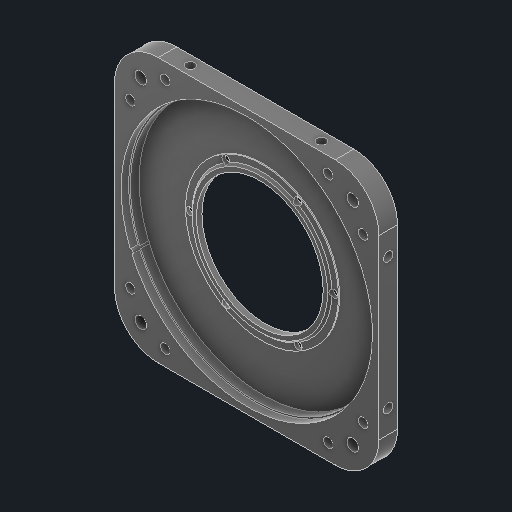
# Autodesk Inventor part: stator_center_01_back_p
Saved by Autodesk Inventor 2026.1 (Build 301233000, 233)
## iProperties
Created: 2026-04-12
Part Number: stator_center_01_back_p
Material: PC/ABS Plastic
Document SubType Name: Modeling
Designer: aaron
Density: 1.1 g/cm^3
Appearance: Smooth - White
Author: aaron
Autodesk Inventor part; units mm, degrees
ref_plane "YZ Plane" through (0, 0, 0) normal (1, 0, 0) x (0, 1, 0)
ref_plane "XZ Plane" through (0, 0, 0) normal (0, 1, 0) x (-1, 0, 0)
ref_plane "XY Plane" through (0, 0, 0) normal (0, 0, 1) x (1, 0, 0)
sketch "Sketch1" plane through (0, 0, 0) normal (0, 0, 1) x (1, 0, 0)
  circle A0 centre (0, 0) radius 57.5
  circle A1 centre (0, 0) radius 60.5
  line L0 (-40.5, 60.5) -> (40.5, 60.5)
  line L1 (60.5, 40.5) -> (60.5, -40.5)
  line L2 (40.5, -60.5) -> (-40.5, -60.5)
  line L3 (-60.5, -40.5) -> (-60.5, 40.5)
  arc A2 (-40.5, 60.5) -> (-60.5, 40.5) centre (-40.5, 40.5) ccw
  arc A3 (60.5, 40.5) -> (40.5, 60.5) centre (40.5, 40.5) ccw
  arc A4 (40.5, -60.5) -> (60.5, -40.5) centre (40.5, -40.5) ccw
  arc A5 (-60.5, -40.5) -> (-40.5, -60.5) centre (-40.5, -40.5) ccw
  dimension "d0" = 115
  dimension "d1" = 121
  dimension "d2" = 20
  constraints: 12 tangent, 8 end point, 8 point on circle, 6 centre point, 3 equal radius, 2 coincident, 2 parallel, 1 horizontal, 1 perpendicular
  measures "d0" diameter of A0
  measures "d1" diameter of A1
  measures "d2" radius of A2
extrude "Extrusion1" add sketch "Sketch1" along normal blind 7.5
sketch "Sketch3" plane through (0, 0, 7.5) normal (0, 0, 1) x (1, 0, 0)
  circle A0 centre (-48.4934, -48.5066) radius 2.65 projected
  circle A1 centre (-37.2752, -53.25) radius 2.15 projected
  circle A2 centre (-53.2398, -37.2897) radius 2.15 projected
  circle A3 centre (-53.25, 37.2752) radius 2.15 projected
  circle A4 centre (-48.5066, 48.4934) radius 2.65 projected
  circle A5 centre (-37.2897, 53.2398) radius 2.15 projected
  circle A6 centre (53.2398, 37.2897) radius 2.15 projected
  circle A7 centre (48.4934, 48.5066) radius 2.65 projected
  circle A8 centre (37.2752, 53.25) radius 2.15 projected
  circle A9 centre (53.25, -37.2752) radius 2.15 projected
  circle A10 centre (48.5066, -48.4934) radius 2.65 projected
  circle A11 centre (37.2897, -53.2398) radius 2.15 projected
  point P0 (0, 0)
extrude "Extrusion3" cut sketch "Sketch3" against normal through all
sketch "Sketch4" plane through (0, 0, 0) normal (0, 0, -1) x (-1, 0, 0)
  circle A0 centre (53.2398, -37.2897) radius 2.15 projected
  circle A1 centre (-53.2398, 37.2897) radius 2.15 projected
  circle A2 centre (-48.5066, -48.4934) radius 2.65 projected
  circle A3 centre (-37.2897, -53.2398) radius 2.15 projected
  circle A4 centre (37.2897, 53.2398) radius 2.15 projected
  circle A5 centre (48.4934, -48.5066) radius 2.65 projected
  circle A6 centre (53.25, 37.2752) radius 2.15 projected
  circle A7 centre (-48.4934, 48.5066) radius 2.65 projected
  circle A8 centre (-53.25, -37.2752) radius 2.15 projected
  circle A9 centre (-37.2752, 53.25) radius 2.15 projected
  circle A10 centre (48.5066, 48.4934) radius 2.65 projected
  circle A11 centre (37.2752, -53.25) radius 2.15 projected
  line L0 (60.5, 40.5) -> (60.5, -40.5) projected
  arc A12 (60.5, 40.5) -> (40.5, 60.5) centre (40.5, 40.5) ccw projected
  line L1 (-40.5, 60.5) -> (40.5, 60.5) projected
  arc A13 (-40.5, 60.5) -> (-60.5, 40.5) centre (-40.5, 40.5) ccw projected
  line L2 (-60.5, -40.5) -> (-60.5, 40.5) projected
  arc A14 (-60.5, -40.5) -> (-40.5, -60.5) centre (-40.5, -40.5) ccw projected
  line L3 (40.5, -60.5) -> (-40.5, -60.5) projected
  arc A15 (40.5, -60.5) -> (60.5, -40.5) centre (40.5, -40.5) ccw projected
  circle A16 centre (0, 0) radius 57.5 projected
  circle A17 centre (0, 0) radius 29
  dimension "d28" = 58
  constraints: 1 centre point, 1 coincident
  measures "d28" diameter of A17
extrude "Extrusion4" add sketch "Sketch4" along normal blind 1 contours L0 A15 L3 A14 L2 A13 L1 A12 | A16
sketch "Sketch5" plane through (0, 0, 0) normal (0, 0, 1) x (1, 0, 0)
  circle A0 centre (0, 0) radius 57.5 projected
  circle A1 centre (0, 0) radius 56.75
  dimension "d31" = 113.5
  constraints: 1 centre point, 1 coincident
  measures "d31" diameter of A1
extrude "Extrusion5" add sketch "Sketch5" along normal blind 4
sketch "Sketch6" plane through (0, 0, 0) normal (0, 0, 1) x (1, 0, 0)
  circle A0 centre (0, 0) radius 29 projected
  circle A1 centre (0, 0) radius 35
  dimension "d34" = 6
  constraints: 1 centre point
  measures "d34" radial gap between concentric circles of A0 A1
extrude "Extrusion6" add sketch "Sketch6" along normal blind 0.5
sketch "Sketch7" plane through (0, 0, 0.5) normal (0, 0, 1) x (1, 0, 0)
  circle A0 centre (0, 0) radius 29 projected
  circle A1 centre (0, 0) radius 31
  dimension "d37" = 2
  constraints: 1 centre point
  measures "d37" radial gap between concentric circles of A0 A1
extrude "Extrusion7" add sketch "Sketch7" along normal blind 1
chamfer "Chamfer1" distance 1 angle 45 1 edges at (-31, 0, 0.5)
sketch "Sketch8" plane through (0, 0, -1) normal (0, 0, -1) x (-1, 0, 0)
  circle A0 centre (32.9998, -0.1078) radius 1.65 projected
  circle A1 centre (0, 0) radius 29 projected
  circle A2 centre (32.9998, -0.1078) radius 1.75
  circle A3 centre (16.5932, 28.5248) radius 1.75
  circle A4 centre (-16.4066, 28.6326) radius 1.75
  circle A5 centre (-32.9998, 0.1078) radius 1.75
  circle A6 centre (-16.5932, -28.5248) radius 1.75
  circle A7 centre (16.4066, -28.6326) radius 1.75
  point P0 (0, 0)
  dimension "d43" = 3.5
  dimension "d46" = 360
  constraints: 6 centre point, 1 coincident, 13 other
  measures "d43" diameter of A2
extrude "Extrusion8" cut sketch "Sketch8" against normal through all contours A0 | A2 | A3 | A4 | A5 | A6 | A7
sketch "Sketch10" plane through (0, 0, 7.5) normal (0, 0, 1) x (1, 0, 0)
  arc A0 (-52.5046, -23.4417) -> (-51.9843, -22.1333) centre (-52.9044, -22.525) ccw projected
  arc A1 (-51.9843, -22.1333) -> (-53.2881, -21.6016) centre (-52.9044, -22.525) ccw projected
  circle A2 centre (-52.9044, -22.525) radius 0.9
  point P0 (0, 0)
  dimension "d50" = 1.8
  constraints: 1 centre point, 1 coincident
  measures "d50" diameter of A2
extrude "Extrusion9" add sketch "Sketch10" against normal up to surface (7.5 mm away)
sketch "Sketch11" plane through (-40.5, 60.5, 7.5) normal (0, 1, 0) x (1, 0, 0)
  line L0 (5.3603, 0) -> (5.3603, 8.5) projected
  line L1 (75.6252, 0) -> (75.6252, 8.5) projected
  circle A0 centre (40.5, 4.25) radius 2.15
  line L2 (101, 8.5) -> (101, 0) projected
  line L3 (-20, 0) -> (-20, 8.5) projected
  line L4 (-20, 0) -> (0, 0) projected
  line L5 (0, 8.5) -> (-20, 8.5) projected
  circle A1 centre (10.5, 4.25) radius 2.15
  circle A2 centre (70.5, 4.25) radius 2.15
  point P0 (40.5, 7.5)
  dimension "d53" = 4.3
  dimension "d54" = 121
  dimension "d55" = 8.5
  dimension "d56" = 60.5
  dimension "d57" = 4.25
  dimension "d60" = 30
  dimension "d67" = 30
  constraints: 3 centre point, 2 horizontal, 4 other
  measures "d53" diameter of A0
  measures "d54" distance between parallel lines of L2 L3
  measures "d55" distance between parallel lines of L4 L5
  measures "d56" distance from line of L3 A0.centre
  measures "d57" distance from line of L5 A0.centre
  measures "d60" distance of A0.centre A1.centre
  measures "d67" distance of A0.centre A2.centre
extrude "Extrusion10" cut sketch "Sketch11" against normal blind 10 contours A1 | A2
sketch "Sketch12" plane through (-40.5, -60.5, 7.5) normal (0, -1, 0) x (1, 0, 0)
  circle A0 centre (10.5, -4.25) radius 2.15 projected
  circle A1 centre (70.5, -4.25) radius 2.15 projected
  point P0 (40.5, -7.5)
extrude "Extrusion11" cut sketch "Sketch12" against normal blind 10
sketch "Sketch13" plane through (-60.5, -40.5, 7.5) normal (-1, 0, 0) x (0, 0, 1)
  line L0 (-8.5, -20) -> (0, -20) projected
  line L1 (-8.5, 101) -> (0, 101) projected
  line L2 (-8.5, 101) -> (-8.5, 81) projected
  line L3 (0, 81) -> (0, 101) projected
  circle A0 centre (-4.25, 70.5) radius 2.15
  circle A1 centre (-4.25, 10.5) radius 2.15
  point P0 (-7.5, 40.5)
  dimension "d76" = 121
  dimension "d77" = 8.5
  dimension "d78" = 4.3
  dimension "d79" = 30.5
  dimension "d80" = 4.25
  dimension "d83" = 60
  constraints: 2 centre point, 1 vertical, 2 other
  measures "d76" distance between parallel lines of L0 L1
  measures "d77" distance between parallel lines of L2 L3
  measures "d78" diameter of A0
  measures "d79" distance from line of L1 A0.centre
  measures "d80" distance from line of L2 A0.centre
  measures "d83" distance of A0.centre A1.centre
extrude "Extrusion12" cut sketch "Sketch13" against normal blind 10
sketch "Sketch14" plane through (60.5, -40.5, 7.5) normal (1, 0, 0) x (0, 0, -1)
  circle A0 centre (4.25, 70.5) radius 2.15 projected
  circle A1 centre (4.25, 10.5) radius 2.15 projected
  point P0 (7.5, 40.5)
extrude "Extrusion13" cut sketch "Sketch14" against normal blind 10
equation "\"d56\" = 0.5 * d54"
equation "\"d57\" = 0.5 * d55"
equation "\"d67\" = d60"
equation "\"d80\" = 0.5 * d77"
body "Solid1"
